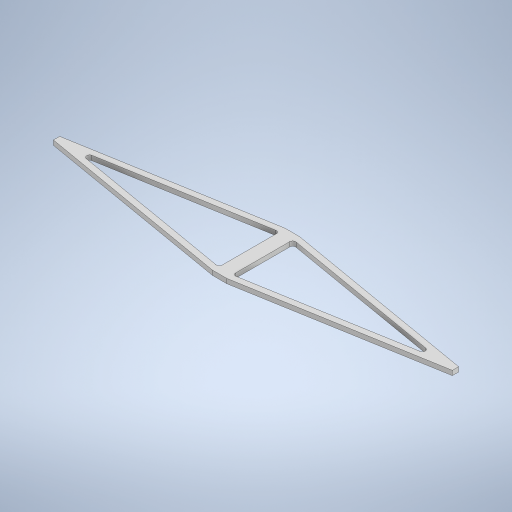
# Autodesk Inventor part: Main Support
Saved by Autodesk Inventor 2023 (Build 270158000, 158)
## iProperties
Created: 2023-03-16
Part Number: Main Support
Material: Generic
Document SubType Name: Modeling
Designer: bugme
Density: 1 g/cm^3
Appearance: Default
Author: bugme
Autodesk Inventor part; units mm, degrees
ref_plane "YZ Plane" through (0, 0, 0) normal (1, 0, 0) x (0, 1, 0)
ref_plane "XZ Plane" through (0, 0, 0) normal (0, 1, 0) x (-1, 0, 0)
ref_plane "XY Plane" through (0, 0, 0) normal (0, 0, 1) x (1, 0, 0)
sketch "Sketch1" plane through (0, 0, 0) normal (0, 1, 0) x (-1, 0, 0)
  line L0 (420, 0) -> (-420, 0) projected
  line L1 (0, 50) -> (-10, 50)
  line L2 (0, -50) -> (-10, -50)
  line L3 (-10, -50) -> (-300, 0)
  line L4 (-300, 0) -> (-10, 50)
  line L5 (0, 50) -> (0, -50)
  line L6 (0, 50) -> (10, 50)
  line L7 (0, -50) -> (10, -50)
  line L8 (10, -50) -> (300, 0)
  line L9 (300, 0) -> (10, 50)
  line L10 (-300, 0) -> (300, 0)
  line L11 (0, -70) -> (0, 70) projected
  line L12 (-300, 0) -> (-300, 0)
  line L13 (300, 0) -> (300, 0)
  line L14 (0, 42) -> (9.3154, 42)
  line L15 (9.3154, 42) -> (252.9154, 0)
  line L16 (252.9154, 0) -> (9.3154, -42)
  line L17 (9.3154, -42) -> (0, -42)
  line L18 (0, 42) -> (-9.3154, 42)
  line L19 (-9.3154, 42) -> (-252.9154, 0)
  line L20 (-252.9154, 0) -> (-9.3154, -42)
  line L21 (-9.3154, -42) -> (0, -42)
  line L22 (9.3154, 42) -> (9.3154, -42)
  line L23 (-9.3154, 42) -> (-9.3154, -42)
  point P0 (0, 0)
  point P1 (300, 0)
  point P2 (-300, 0)
  dimension "d36" = 600
  dimension "d38" = 10
  dimension "d39" = 100
  dimension "d44" = 8
  dimension "d45" = 8
  dimension "d47" = 600
  dimension "d49" = 300
  dimension "d51" = 0
  dimension "d52" = 300
  dimension "d53" = 300
  dimension "d54" = 0
  dimension "d55" = 0
  dimension "d56" = 0
  dimension "d57" = 0
  dimension "d60" = 0
  constraints: 44 end point, 5 symmetric about line, 4 vertical, 3 parallel, 2 point on line, 1 horizontal, 6 other
  measures "d36" distance of point (-300, 0) point (300, 0)
  measures "d38" distance of L1.start L1.end
  measures "d39" distance of L1.start L2.start
  measures "d44" distance between parallel lines of L8 L16
  measures "d45" distance between parallel lines of L4 L19
  measures "d47" distance between parallel lines of L12 L13
  measures "d49" distance between parallel lines of L11 L13
  measures "d51" distance from line of point (300, 0) L0
  measures "d52" distance from line of point (300, 0) L11
  measures "d53" distance from line of L10.end L11
  measures "d54" distance from line of L18.start L11
  measures "d55" distance from line of L14.start L11
  measures "d56" distance from line of L21.end L11
  measures "d57" distance from line of L17.end L11
  measures "d60" distance from line of point (-300, 0) L0
extrude "Main_block" add sketch "Sketch1" along normal blind 6.35 contours L8 L7 L5 L17 L16 L0 | L0 L15 L14 L5 L6 L9 | L22 L17 L5 L0 | L0 L5 L14 L22 | L2 L3 L0 L20 L21 L5 | L5 L18 L19 L0 L4 L1 | L5 L21 L23 L0 | L0 L23 L18 L5
fillet "Fillet7" radius 4 6 edges at (-9.3154, 3.175, -42) (9.3154, 3.175, -42) (9.3154, 3.175, 42) (-9.3154, 3.175, 42) (252.9154, 3.175, 0) (-252.9154, 3.175, 0)
sketch "Sketch4" plane through (0, 6.35, 0) normal (0, 1, 0) x (1, 0, 0)
  line L0 (-300, 0) -> (-10, -50) projected
  line L1 (-10, 50) -> (-300, 0) projected
  line L2 (-275, 4.3103) -> (-275, -4.3103)
  line L3 (-275, -4.3103) -> (-300, 0)
  line L4 (-300, 0) -> (-275, 4.3103)
  line L5 (0, 70) -> (0, -70) projected
  line L6 (275, 4.3103) -> (275, -4.3103)
  line L7 (275, -4.3103) -> (300, 0)
  line L8 (300, 0) -> (275, 4.3103)
  point P0 (0, 0)
  constraints: 12 end point, 3 symmetric about line, 2 point on line, 1 vertical
extrude "Extrusion4" cut sketch "Sketch4" against normal blind 10
body "Solid1"
